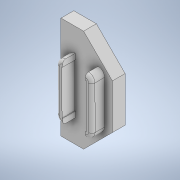
# Autodesk Inventor part: Servo Holder Module
Saved by Autodesk Inventor 2020.2 (Build 242310000, 310)
## iProperties
Created: 2020-03-03
Part Number: Servo Holder Module
Material: Generic
Document SubType Name: Modeling
Designer: Varun Kumar
Density: 1 g/cm^3
Appearance: Default
Author: Varun Kumar
Autodesk Inventor part; units mm, degrees
ref_plane "YZ Plane" through (0, 0, 0) normal (1, 0, 0) x (0, 1, 0)
ref_plane "XZ Plane" through (0, 0, 0) normal (0, 1, 0) x (-1, 0, 0)
ref_plane "XY Plane" through (0, 0, 0) normal (0, 0, 1) x (1, 0, 0)
sketch "Sketch1" plane through (0, 0, 0) normal (0, 0, 1) x (1, 0, 0)
  line L0 (-38.1, -25.4) -> (38.1, -25.4)
  line L1 (38.1, -25.4) -> (38.1, 25.4)
  line L2 (38.1, 25.4) -> (-38.1, 25.4)
  line L3 (-38.1, 25.4) -> (-38.1, -25.4)
  line L4 (-38.1, -25.4) -> (38.1, 25.4) construction
  line L5 (38.1, -25.4) -> (-38.1, 25.4) construction
  point P0 (0, 0)
  dimension "d0" = 76.2
  dimension "d1" = 50.8
  constraints: 12 end point, 2 midpoint, 2 parallel, 1 horizontal, 1 perpendicular
  measures "d0" distance of L2.end L1.end
  measures "d1" distance of L1.end L0.end
extrude "Extrusion1" add sketch "Sketch1" along normal blind 6.35
sketch "Sketch2" plane through (0, 0, 6.35) normal (0, 0, 1) x (1, 0, 0)
  line L0 (5.6355, 11.0158) -> (5.6275, 13.857)
  line L1 (5.9693, 11.0167) -> (5.6355, 11.0158)
  arc A0 (8.8114, 10.6909) -> (5.6275, 13.857) centre (5.6364, 10.682) ccw
  line L2 (8.8114, 10.6909) -> (8.871, -10.6415)
  line L3 (6.0307, -10.9832) -> (5.9693, 11.0167)
  line L4 (-6.0307, 10.9832) -> (-5.9693, -11.0167)
  line L5 (-6.0307, 10.9832) -> (-5.9693, -11.0167)
  line L6 (-5.9693, -11.0167) -> (-5.6355, -11.0158)
  line L7 (-5.6355, -11.0158) -> (-5.9693, -11.0167)
  arc A1 (-8.8114, -10.6909) -> (-5.6275, -13.857) centre (-5.6364, -10.682) ccw
  arc A2 (-8.8114, -10.6909) -> (-5.6275, -13.857) centre (-5.6364, -10.682) ccw
  line L8 (-5.6969, 10.9841) -> (-6.0307, 10.9832)
  line L9 (-5.7048, 13.8253) -> (-5.6969, 10.9841)
  arc A3 (-5.7048, 13.8253) -> (-8.871, 10.6415) centre (-5.696, 10.6504) ccw
  arc A4 (-5.7048, 13.8253) -> (-8.871, 10.6415) centre (-5.696, 10.6504) ccw
  line L10 (5.6969, -10.9841) -> (6.0307, -10.9832)
  arc A5 (5.7048, -13.8253) -> (8.871, -10.6415) centre (5.696, -10.6504) ccw
  line L11 (5.7048, -13.8253) -> (5.6969, -10.9841)
  line L12 (-5.6355, -11.0158) -> (-5.6275, -13.857)
  line L13 (-5.6355, -11.0158) -> (-5.6275, -13.857)
  line L14 (-8.871, 10.6415) -> (-8.8114, -10.6909)
  line L15 (-8.871, 10.6415) -> (-8.8114, -10.6909)
  line L16 (5.6275, 13.857) -> (-5.6275, -13.857)
  line L17 (8.8412, 0.0247) -> (-8.8412, -0.0247)
  line L18 (0, 0) -> (-0.0387, 13.8412)
  line L19 (-13.078, 0) -> (-13.078, 5.6662)
  point P0 (0, 0)
  point P1 (0, 0)
  point P2 (-5.7048, 13.8253)
  constraints: 40 end point, 12 point on circle, 6 centre point, 5 perpendicular, 3 midpoint, 2 concentric, 1 point on line, 1 tangent, 1 vertical
extrude "Extrusion2" add sketch "Sketch2" along normal blind 6.35 contours L0 A0 L2 L17 L3 L1 | L17 L2 A5 L11 L10 L3 | A1 L14 L17 L4 L6 L12 | L17 L14 A3 L9 L8 L4
fillet "Fillet1" radius 1.5875 6 edges at (8.8412, 0.0247, 12.7) (7.9473, -12.8891, 12.7) (7.8752, 12.9333, 12.7) (-7.8752, -12.9333, 12.7) (-7.9473, 12.8891, 12.7) (-8.8412, -0.0247, 12.7)
sketch "Sketch3" plane through (38.1, -25.4, 0) normal (1, 0, 0) x (0, 0, -1)
  line L0 (0, 0) -> (0, 50.8) projected
  line L1 (0, 50.8) -> (-6.35, 50.8) projected
  line L2 (-6.35, 0) -> (-6.35, 50.8) projected
  line L3 (0, 0) -> (-6.35, 0) projected
  point P0 (0, 25.4)
extrude "Extrusion3" cut sketch "Sketch3" against normal blind 25.4
sketch "Sketch4" plane through (-38.1, -25.4, 0) normal (-1, 0, 0) x (0, 0, 1)
  line L0 (4.925, 17.15) -> (1.425, 17.15)
  line L1 (1.425, 17.15) -> (1.425, 33.65)
  line L2 (1.425, 33.65) -> (4.925, 33.65)
  line L3 (4.925, 33.65) -> (4.925, 17.15)
  line L4 (4.925, 17.15) -> (1.425, 33.65) construction
  line L5 (1.425, 17.15) -> (4.925, 33.65) construction
  point P0 (0, 25.4)
  point P1 (3.175, 25.4)
  dimension "d9" = 3.5
  dimension "d10" = 16.5
  constraints: 12 end point, 2 midpoint, 2 parallel, 1 horizontal, 1 perpendicular
  measures "d9" distance of L1.end L2.end
  measures "d10" distance of L0.end L1.end
extrude "Extrusion4" add sketch "Sketch4" along normal blind 3.302
sketch "Sketch5" plane through (-38.1, -8.25, 4.925) normal (0, 0, 1) x (1, 0, 0)
  line L0 (-3.302, 0) -> (-3.302, 16.5) projected
  line L1 (0, 16.5) -> (0, 0) projected
  line L2 (0, 16.5) -> (-3.302, 16.5) projected
  line L3 (-3.302, 0) -> (-3.302, 16.5) projected
  line L4 (0, 0) -> (-3.302, 0) projected
  line L5 (-3.302, 16.5) -> (-3.175, 16.5)
  line L6 (0, 16.5) -> (-3.302, 16.5) projected
  line L7 (-3.175, 16.5) -> (-3.175, 16.5685)
  line L8 (-3.302, 16.5) -> (-3.302, 0) projected
  line L9 (-3.175, 16.5685) -> (-3.302, 16.5)
  point P0 (38.1, 8.25)
  point P1 (-3.175, 16.5)
  dimension "d13" = 0.127
  constraints: 6 end point, 1 perpendicular, 1 point on line
  measures "d13" distance of L2.end L5.end
sketch3d "3D Sketch1"
  line L0 (-41.402, 8.25, 4.925) -> (-41.402, 8.25, 1.425)
  line L1 (-41.402, 8.25, 1.425) -> (-41.402, -8.25, 1.425)
  line L2 (-41.402, -8.25, 1.425) -> (-41.402, -8.25, 4.925)
  line L3 (-41.402, -8.25, 4.925) -> (-41.402, 8.25, 4.925)
sweep "Sweep1" add profiles "Sketch5" path "3D Sketch1" contours L9 L7 L2
chamfer "Chamfer1" distance 14.2875 angle 45 4 edges at (-38.1, -25.4, 3.175) (-38.1, 25.4, 3.175) (12.7, -25.4, 3.175) (12.7, 25.4, 3.175)
sketch "Sketch6" plane through (-41.402, -25.4, 0) normal (-1, 0, 0) x (0, 0, 1)
  line L0 (-26.5368, -66.9991) -> (26.5368, -66.9991)
  line L1 (26.5368, -66.9991) -> (26.5368, 66.9991)
  line L2 (26.5368, 66.9991) -> (-26.5368, 66.9991)
  line L3 (-26.5368, 66.9991) -> (-26.5368, -66.9991)
  line L4 (0, 0) -> (6.35, 0) projected
  line L5 (-26.5368, -66.9991) -> (26.5368, 66.9991) construction
  line L6 (26.5368, -66.9991) -> (-26.5368, 66.9991) construction
  point P0 (0, 25.4)
  constraints: 12 end point, 2 midpoint, 2 parallel, 1 horizontal, 1 perpendicular
extrude "Extrusion5" cut sketch "Sketch6" against normal blind 28.575
sketch "Sketch7" plane through (0, 0, 0) normal (0, 0, -1) x (-1, 0, 0)
  line L0 (-8.025, 1.675) -> (-8.025, -1.675)
  line L1 (-8.025, -1.675) -> (8.025, -1.675)
  line L2 (8.025, -1.675) -> (8.025, 1.675)
  line L3 (8.025, 1.675) -> (-8.025, 1.675)
  line L4 (-8.025, 1.675) -> (8.025, -1.675) construction
  line L5 (-8.025, -1.675) -> (8.025, 1.675) construction
  line L6 (0, 3.175) -> (0, -3.175)
  point P0 (0, 0)
  point P1 (0, 0)
  dimension "d21" = 3.35
  dimension "d22" = 16.05
  constraints: 14 end point, 2 parallel, 1 midpoint, 1 perpendicular
  measures "d21" distance of L2.end L1.end
  measures "d22" distance of L1.end L0.end
extrude "Extrusion6" add sketch "Sketch7" along normal blind 3.302
sketch "Sketch8" plane through (-8.025, 1.675, 0) normal (0, 1, 0) x (0, 0, 1)
  line L0 (-3.302, 16.05) -> (-3.302, 0) projected
  line L1 (-3.302, 16.05) -> (-3.175, 16.05)
  line L2 (0, 16.05) -> (-3.302, 16.05) projected
  line L3 (-3.175, 16.05) -> (-3.175, 16.1358)
  line L4 (-3.175, 16.1358) -> (-3.302, 16.05)
  point P0 (0, 8.025)
  dimension "d25" = 0.127
  constraints: 6 end point, 1 perpendicular, 1 point on line
  measures "d25" distance of L0.start L1.end
sketch3d "3D Sketch2"
  line L0 (8.025, 1.675, -3.302) -> (8.025, -1.675, -3.302)
  line L1 (8.025, -1.675, -3.302) -> (-8.025, -1.675, -3.302)
  line L2 (-8.025, -1.675, -3.302) -> (-8.025, 1.675, -3.302)
  line L3 (-8.025, 1.675, -3.302) -> (8.025, 1.675, -3.302)
sweep "Sweep2" add profiles "Sketch8" path "3D Sketch2"
body "Solid1"
